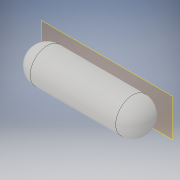
# Autodesk Inventor part: P1704_003_mainDroite
Saved by Autodesk Inventor 2019 (Build 230136000, 136)
## iProperties
Created: 2019-04-29
Part Number: P1704_003_mainDroite
Material: Générique
Document SubType Name: Modeling
Designer: Joan.MAILLARD
Density: 1 g/cm^3
Appearance: Par défaut
Author: Joan.MAILLARD
Autodesk Inventor part; units mm, degrees
ref_plane "YZ Plane" through (0, 0, 0) normal (1, 0, 0) x (0, 1, 0)
ref_plane "XZ Plane" through (0, 0, 0) normal (0, 1, 0) x (-1, 0, 0)
sketch "Esquisse1" plane through (0, 0, 0) normal (0, 1, 0) x (-1, 0, 0)
  line L0 (0, 0) -> (-150, 0)
  line L1 (-150, 0) -> (-150, -30)
  line L2 (-150, -30) -> (0, -30)
  line L3 (0, -30) -> (0, 0)
  arc A0 (0, -30) -> (30, 0) centre (0, 0) ccw
  line L4 (30, 0) -> (0, 0)
  line L5 (0, 0) -> (0, -30)
  line L6 (-150, 0) -> (-150, -30)
  arc A1 (-180, 0) -> (-150, -30) centre (-150, 0) ccw
  line L7 (-150, 0) -> (-180, 0)
  dimension "d1" = 30
  dimension "d2" = 150
  constraints: 16 end point, 4 line through centre, 4 point on circle, 3 equal length, 2 centre point, 2 coincident, 2 horizontal, 2 perpendicular, 1 vertical
  measures "d1" distance of L2.end L0.start
  measures "d2" distance of L1.end L2.end
revolve "Révolution1" add sketch "Esquisse1" angle 360 about axis through (0, 0, 0) along (1, 0, 0)
ref_plane "Plan de construction1" through (75, 0, -30) normal (0, 0, 1) x (1, 0, 0)
sketch "Esquisse2" plane through (75, 0, -30) normal (0, 0, 1) x (1, 0, 0)
  line L0 (-75, 0) -> (-105, 0)
  line L1 (-105, 0) -> (-105, -30)
  line L2 (-105, -30) -> (-75, -30)
  line L3 (-75, -30) -> (-75, 0)
  dimension "d4" = 30
  dimension "d5" = 30
  constraints: 8 end point, 2 parallel, 1 horizontal, 1 perpendicular
  measures "d4" distance of L0.start L0.end
  measures "d5" distance of L2.end L0.start
extrude "Extrusion1" cut sketch "Esquisse2" along normal blind 30
